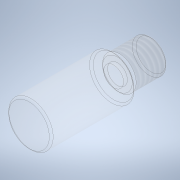
# Autodesk Inventor part: Glas
Saved by Autodesk Inventor 2021.3 (Build 253353000, 353)
## iProperties
Created: 2021-10-18
Part Number: Glas
Material: Generisch
Document SubType Name: Modeling
Designer: bhelg
Density: 1 g/cm^3
Appearance: Klar - hell
Author: bhelg
Autodesk Inventor part; units mm, degrees
ref_plane "YZ Plane" through (0, 0, 0) normal (1, 0, 0) x (0, 1, 0)
ref_plane "XZ Plane" through (0, 0, 0) normal (0, 1, 0) x (-1, 0, 0)
ref_plane "XY Plane" through (0, 0, 0) normal (0, 0, 1) x (1, 0, 0)
sketch "Skizze1" plane through (0, 0, 0) normal (0, 1, 0) x (-1, 0, 0)
  line L0 (0, 0) -> (5.775, 0)
  line L1 (5.775, 0) -> (5.775, -22)
  line L2 (5.775, -22) -> (2.075, -22)
  line L3 (2.075, -22) -> (2.075, -23)
  line L4 (2.075, -23) -> (4.35, -23)
  line L5 (4.35, -23) -> (4.35, -31.7)
  line L6 (4.35, -31.7) -> (0, -31.7)
  line L7 (0, -31.7) -> (0, 0)
  dimension "d0" = 5.775
  dimension "d1" = 22
  dimension "d2" = 3.7
  dimension "d3" = 1
  dimension "d4" = 8.7
  dimension "d5" = 4.35
  constraints: 16 end point, 7 perpendicular, 1 horizontal
  measures "d0" distance of L0.start L0.end
  measures "d1" distance of L0.end L1.end
  measures "d2" distance of L1.end L2.end
  measures "d3" distance of L2.end L3.end
  measures "d4" distance of L4.end L5.end
  measures "d5" distance between parallel lines of L5 L7
revolve "Umdrehung1" add sketch "Skizze1" angle 360 about axis through (0, 0, -31.7) along (0, 0, 1)
fillet "Rundung1" radius 0.5 6 edges at (5.775, 0, -22) (5.775, 0, 0) (4.35, 0, -23) (4.35, 0, -31.7) (2.075, 0, -22) (2.075, 0, -23)
thread "Gewinde1" size "M9x1.25" class "6g" standard "ANSI Metric M Profile" full length
